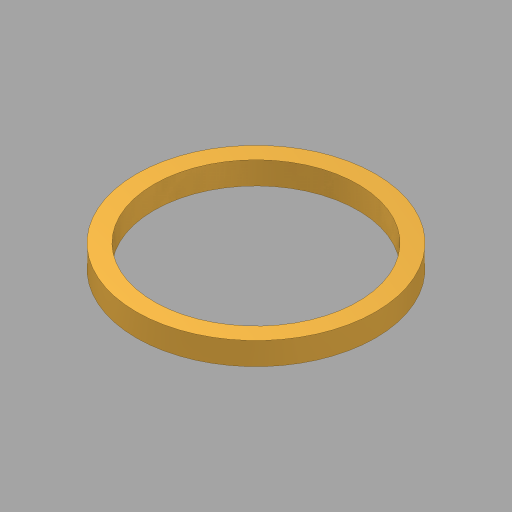
# Autodesk Inventor part: press
Saved by Autodesk Inventor 2024 (Build 280153020, 153B)
## iProperties
Created: 2023-11-04
Part Number: press
Material: Brass, Soft Yellow
Document SubType Name: Modeling
Designer: schanen
Density: 8.47 g/cm^3
Appearance: Brass - Satin
Mass: 25.7844 g
Surface Area: 27.3978 cm^2
Volume: 3.0442 cm^3
Author: schanen
Autodesk Inventor part; units mm, degrees
ref_plane "YZ Plane" through (0, 0, 0) normal (1, 0, 0) x (0, 1, 0)
ref_plane "XZ Plane" through (0, 0, 0) normal (0, 1, 0) x (-1, 0, 0)
ref_plane "XY Plane" through (0, 0, 0) normal (0, 0, 1) x (1, 0, 0)
sketch "Sketch1" plane through (0, 0, 0) normal (0, 0, 1) x (1, 0, 0)
  line L0 (-22.5, 0) -> (-26.4, 0)
  line L1 (-26.4, 0) -> (-26.4, 5)
  line L2 (-26.4, 5) -> (-22.5, 5)
  line L3 (-22.5, 5) -> (-22.5, 0)
  line L4 (0, -1) -> (0, 6) projected
  point P0 (0, 0)
  dimension "d0" = 22.5
  dimension "d1" = 5
  dimension "d2" = 3.9
  constraints: 8 end point, 2 parallel, 1 horizontal, 1 horizontal alignment, 1 perpendicular
  measures "d0" distance from line of point (0, 0) L3
  measures "d1" distance of L2.end L0.start
  measures "d2" distance of L1.end L2.end
revolve "Revolution1" add sketch "Sketch1" angle 360 about axis through (0, -10, 0) along (0, 1, 0)
equation "\"d0\" = 0.5 * oring_id"
equation "\"oring_id\" = 45"
body "Solid1"
